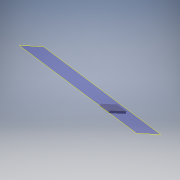
# Autodesk Inventor part: 베어링받침대2
Saved by Autodesk Inventor 2017 (Build 210142000, 142)
## iProperties
Part Number: 베어링받침대2
Material: 일반
Document SubType Name: Modeling
Designer: minom
Density: 1 g/cm^3
Appearance: 기본값
Author: minom
Autodesk Inventor part; units mm, degrees
ref_plane "YZ Plane" through (0, 0, 0) normal (1, 0, 0) x (0, 1, 0)
ref_plane "XZ Plane" through (0, 0, 0) normal (0, 1, 0) x (-1, 0, 0)
ref_plane "XY Plane" through (0, 0, 0) normal (0, 0, 1) x (1, 0, 0)
ref_plane "작업 평면1" through (-100.0158, 30.7128, 83.3729) normal (-0.0776, -0.4451, -0.8921) x (0.0684, 0.8904, -0.4501)
sketch "스케치1" plane through (-100.0158, 30.7128, 83.3729) normal (-0.0776, -0.4451, -0.8921) x (0.0684, 0.8904, -0.4501)
  line L0 (3, -48) -> (45, -48)
  line L1 (45, -48) -> (45, -72)
  line L2 (45, -72) -> (3, -72)
  line L3 (3, -72) -> (3, -48)
  point P0 (17.0185, 105.6505)
  dimension "d6" = 42
  dimension "d7" = 24
  constraints: 8 end point, 2 parallel, 1 horizontal, 1 perpendicular
  measures "d6" distance of L1.end L2.end
  measures "d7" distance of L0.end L1.end
extrude "돌출1" add sketch "스케치1" along normal blind 5
